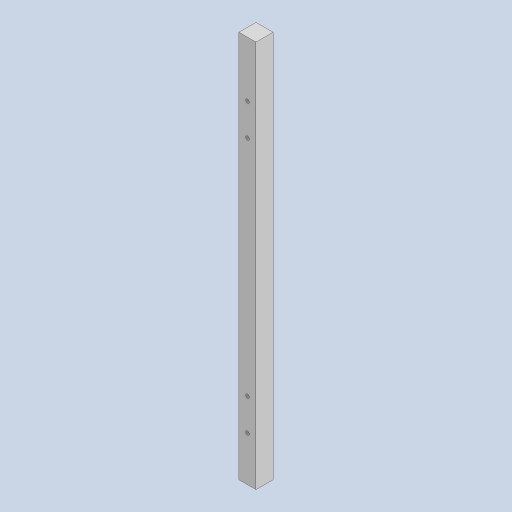
# Autodesk Inventor part: Long side frame
Saved by Autodesk Inventor 2023.4 (Build 274418000, 418)
## iProperties
Created: 2024-02-06
Part Number: Long side frame
Material: Generic
Document SubType Name: Modeling
Designer: PalumaCMM
Density: 1 g/cm^3
Appearance: Default
Author: PalumaCMM
Autodesk Inventor part; units mm, degrees
ref_plane "YZ Plane" through (0, 0, 0) normal (1, 0, 0) x (0, 1, 0)
ref_plane "XZ Plane" through (0, 0, 0) normal (0, 1, 0) x (-1, 0, 0)
ref_plane "XY Plane" through (0, 0, 0) normal (0, 0, 1) x (1, 0, 0)
sketch "Sketch1" plane through (0, 0, 0) normal (0, 0, 1) x (1, 0, 0)
  line L0 (0, 0) -> (40, 0)
  line L1 (40, 0) -> (40, 910)
  line L2 (40, 910) -> (0, 910)
  line L3 (0, 910) -> (0, 0)
  dimension "d0" = 40
  dimension "d1" = 910
  constraints: 8 end point, 2 parallel, 1 horizontal, 1 perpendicular
  measures "d0" distance of L2.end L1.end
  measures "d1" distance of L1.end L0.end
extrude "Extrusion1" add sketch "Sketch1" along normal blind 40
sketch "Sketch2" plane through (0, 0, 40) normal (0, 0, 1) x (1, 0, 0)
  line L0 (40, 910) -> (0, 910) projected
  line L1 (0, 0) -> (40, 0) projected
  line L2 (0, 910) -> (0, 0) projected
  line L3 (40, 0) -> (40, 910) projected
  point P0 (20, 780)
  point P1 (20, 105)
  point P2 (20, 180)
  point P3 (20, 910)
  point P4 (20, 0)
  point P5 (20, 705)
  point P6 (20, 630)
  point P7 (20, 555)
  point P8 (20, 480)
  point P9 (20, 405)
  point P10 (20, 330)
  point P11 (20, 255)
  dimension "d4" = 130
  dimension "d5" = 105
  dimension "d6" = 20
  dimension "d7" = 40
  dimension "d8" = 20
  dimension "d9" = 75
  dimension "d10" = 20
  dimension "d11" = 75
  dimension "d12" = 20
  dimension "d13" = 75
  dimension "d14" = 20
  dimension "d15" = 75
  dimension "d16" = 20
  dimension "d17" = 75
  dimension "d18" = 20
  dimension "d19" = 75
  dimension "d20" = 20
  dimension "d21" = 75
  dimension "d22" = 20
  dimension "d23" = 75
  dimension "d24" = 20
  dimension "d25" = 75
  constraints: 2 midpoint
  measures "d4" distance of point (20, 910) point (20, 780)
  measures "d5" distance of point (20, 0) point (20, 105)
  measures "d6" distance from line of L2 point (20, 105)
  measures "d7" distance between parallel lines of L2 L3
  measures "d8" distance from line of L2 point (20, 780)
  measures "d9" distance of point (20, 780) point (20, 705)
  measures "d10" distance from line of L2 point (20, 705)
  measures "d11" distance of point (20, 105) point (20, 180)
  measures "d12" distance from line of L2 point (20, 180)
  measures "d13" distance of point (20, 705) point (20, 630)
  measures "d14" distance from line of L2 point (20, 630)
  measures "d15" distance of point (20, 630) point (20, 555)
  measures "d16" distance from line of L2 point (20, 555)
  measures "d17" distance of point (20, 555) point (20, 480)
  measures "d18" distance from line of L2 point (20, 480)
  measures "d19" distance of point (20, 480) point (20, 405)
  measures "d20" distance from line of L2 point (20, 405)
  measures "d21" distance of point (20, 405) point (20, 330)
  measures "d22" distance from line of L2 point (20, 330)
  measures "d23" distance of point (20, 330) point (20, 255)
  measures "d24" distance from line of L2 point (20, 255)
  measures "d25" distance of point (20, 255) point (20, 180)
hole "Hole1" at (20, 105, 40) at (20, 780, 40) at (20, 705, 40) at (20, 180, 40) direction (0, 0, -1) diameter 8.376 end through all thread size "M10x1.5" class "6H" standard "ISO Metric profile"
equation "\"d6\" = 0.5 * d7"
equation "\"d8\" = d6"
equation "\"d10\" = d8"
equation "\"d11\" = d9"
equation "\"d12\" = d6"
equation "\"d13\" = d9"
equation "\"d14\" = d10"
equation "\"d15\" = d13"
equation "\"d16\" = d14"
equation "\"d17\" = d15"
equation "\"d18\" = d16"
equation "\"d19\" = d17"
equation "\"d20\" = d18"
equation "\"d21\" = d19"
equation "\"d22\" = d20"
equation "\"d23\" = d21"
equation "\"d24\" = d22"
body "Solid1"
